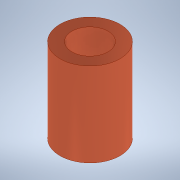
# Autodesk Inventor part: 02_Column25_long
Saved by Autodesk Inventor 2021.1 (Build 251245010, 245A)
## iProperties
Created: 2025-08-17
Part Number: 02_Column25_long
Material: Generic
Document SubType Name: Modeling
Designer: TUAN PC
Density: 1 g/cm^3
Appearance: Metal 1400F Hot
Author: TUAN PC
Autodesk Inventor part; units mm, degrees
ref_plane "YZ Plane" through (0, 0, 0) normal (1, 0, 0) x (0, 1, 0)
ref_plane "XZ Plane" through (0, 0, 0) normal (0, 1, 0) x (-1, 0, 0)
ref_plane "XY Plane" through (0, 0, 0) normal (0, 0, 1) x (1, 0, 0)
sketch "Sketch1" plane through (0, 0, 0) normal (0, 1, 0) x (-1, 0, 0)
  circle A0 centre (0, 0) radius 2.5
  circle A1 centre (0, 0) radius 1.5
  dimension "d0" = 5
  dimension "d1" = 3
  constraints: 2 centre point, 2 coincident
  measures "d0" diameter of A0
  measures "d1" diameter of A1
extrude "Extrusion1" add sketch "Sketch1" along normal blind 7
body "Solid1"
